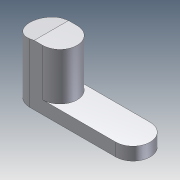
# Autodesk Inventor part: CANH TAY 3
Saved by Autodesk Inventor 2011 (Build 150239000, 239)
## iProperties
Manager: CÁI
Company: TPA
Created: 2018-05-23
Part Number: CANH TAY 3
Material: -
Document SubType Name: Modeling
Designer: hau.np
Surface Area: 955.892 cm^2
Volume: 1437.07 cm^3
Author: hau.np
Comments: GHI CHÚ: 1. DUNG SAI KÍCH THƯỚC GIA CÔNG +/- 0.5 2. LÀM SẠCH BAVIA CẠNH CẮT. 3.
Autodesk Inventor part; units mm, degrees
ref_plane "YZ Plane" through (0, 0, 0) normal (1, 0, 0) x (0, 1, 0)
ref_plane "XZ Plane" through (0, 0, 0) normal (0, 1, 0) x (-1, 0, 0)
ref_plane "XY Plane" through (0, 0, 0) normal (0, 0, 1) x (1, 0, 0)
sketch "Sketch1" plane through (0, 0, 0) normal (0, 0, 1) x (1, 0, 0)
  line L0 (0, 15.9441) -> (0, -15.9441) construction
  line L1 (11.6084, 0) -> (-11.6084, 0) construction
  line L2 (46.4051, 40) -> (246.4051, 40)
  line L3 (246.4051, 40) -> (246.4051, -40)
  line L4 (246.4051, -40) -> (46.4051, -40)
  line L5 (46.4051, -40) -> (46.4051, 40)
  circle A0 centre (46.4051, 0) radius 40
  circle A1 centre (246.4051, 0) radius 40
  point P0 (0, 0)
  point P1 (0, 0)
  dimension "d0" = 80
  dimension "d1" = 200
  constraints: 12 end point, 4 midpoint, 2 horizontal, 2 parallel, 2 vertical alignment, 1 coincident, 1 perpendicular, 1 vertical, 5 other
  measures "d0" distance between parallel lines of L4 L2
  measures "d1" distance from line of L3 point (46.405, 0)
extrude "Extrusion1" add sketch "Sketch1" along normal blind 30
sketch "Sketch2" plane through (0, 0, 30) normal (0, 0, 1) x (1, 0, 0)
  arc A0 (46.4051, 40) -> (46.4051, -40) centre (46.4051, 0) ccw projected
  circle A1 centre (46.4051, 0) radius 40
  line L0 (46.4051, -40) -> (46.4051, 40)
  line L1 (116.4051, 0) -> (76.4051, 0)
  circle A2 centre (76.4051, 0) radius 40
  line L2 (46.4051, 40) -> (76.4051, 40)
  line L3 (76.4051, -40) -> (46.4051, -40)
  point P0 (0, 0)
  constraints: 8 end point, 4 tangent, 3 point on circle, 2 centre point, 2 coincident, 1 parallel, 1 perpendicular
extrude "Extrusion2" add sketch "Sketch2" along normal blind 110
sketch "Sketch3" plane through (46.4051, -40, 0) normal (0, -1, 0) x (1, 0, 0)
  line L0 (-40, 140) -> (0, 140) projected
  line L1 (0, 140) -> (10, 140)
  line L2 (10, 140) -> (-81.693, 123.8321)
  line L3 (-81.693, 123.8321) -> (-81.693, 140)
  line L4 (-81.693, 140) -> (0, 140)
  point P0 (-46.4051, 0)
  constraints: 8 end point, 2 collinear, 1 perpendicular
extrude "Extrusion3" cut sketch "Sketch3" against normal through all
sketch "Sketch4" plane through (0, 0, 0) normal (0, 0, -1) x (-1, 0, 0)
  line L0 (-246.4051, -40) -> (-46.4051, -40) projected
  arc A0 (-46.4051, -40) -> (-46.4051, 40) centre (-46.4051, 0) ccw projected
  line L1 (-46.4051, 40) -> (-246.4051, 40) projected
  arc A1 (-246.4051, 40) -> (-246.4051, -40) centre (-246.4051, 0) ccw projected
  circle A2 centre (-46.4051, 0) radius 8
  point P0 (0, 0)
  constraints: 1 centre point, 1 coincident
extrude "Extrusion4" add sketch "Sketch4" along normal blind 10 contours A2
body "Solid1"
